Autodesk Fusion 360 part; units mm, degrees
(part 4 of 5)
sketch "Boceto5" plane through (0, 0, 0) normal (0, -1, 0) x (1, 0, 0)
  line L0 (-30, -63.3205) -> (-16, -63.3205)
  line L1 (-16, -63.3205) -> (-16, -68.1205)
  line L2 (-16, -68.1205) -> (-30, -68.1205)
  line L3 (-30, -68.1205) -> (-30, -105)
  line L4 (-30, -105) -> (30, -105)
  line L5 (30, -105) -> (30, -68.1205)
  line L6 (30, -68.1205) -> (16, -68.1205)
  line L7 (16, -68.1205) -> (16, -63.3205)
  line L8 (16, -63.3205) -> (30, -63.3205)
  line L9 (30, -63.3205) -> (30, -62.3205)
  arc A0 (32.0096, -54.8205) -> (30, -62.3205) centre (45, -62.3205) ccw
  line L10 (32.0096, -54.8205) -> (56.4434, -12.5)
  arc A1 (69.4338, -5) -> (56.4434, -12.5) centre (69.4338, -20) ccw
  line L11 (69.4338, -5) -> (101.3943, -5)
  arc A2 (107.5227, -7.8577) -> (101.3943, -5) centre (101.3943, -13) ccw
  line L12 (107.5227, -7.8577) -> (126.7013, -30.7139)
  arc A3 (126.7013, -30.7139) -> (130.5315, -32.5) centre (130.5315, -27.5) ccw
  line L13 (130.5315, -32.5) -> (131.95, -32.5)
  line L14 (131.95, -32.5) -> (133.2, -31.25)
  line L15 (133.2, -31.25) -> (133.2, -5)
  line L16 (133.2, -5) -> (138, -5)
  line L17 (138, -5) -> (138, -31.5)
  line L18 (138, -31.5) -> (139, -32.5)
  line L19 (139, -32.5) -> (141.0289, -32.5)
  arc A4 (141.0289, -32.5) -> (149.6891, -17.5) centre (141.0289, -22.5) ccw
  arc A5 (148.5274, 15.3125) -> (149.6891, -17.5) centre (180, 0) ccw
  arc A6 (148.5274, 15.3125) -> (144.0313, 22.5) centre (144.0313, 17.5) ccw
  line L20 (144.0313, 22.5) -> (131.9209, 22.5)
  arc A7 (131.9209, 22.5) -> (125.7926, 19.6423) centre (131.9209, 14.5) ccw
  line L21 (125.7926, 19.6423) -> (115.9041, 7.8577)
  arc A8 (109.7758, 5) -> (115.9041, 7.8577) centre (109.7758, 13) ccw
  line L22 (109.7758, 5) -> (35, 5)
  arc A9 (30, 10) -> (35, 5) centre (35, 10) ccw
  line L23 (30, 10) -> (30, 12.6048)
  arc A10 (30, 12.6048) -> (26.8657, 15.6018) centre (27, 12.6048) ccw
  arc A11 (22.4813, 15.4213) -> (26.8657, 15.6018) centre (0, 615) ccw
  arc A12 (22.4813, 15.4213) -> (22, 14.9217) centre (22.5, 14.9217) ccw
  line L24 (22, 14.9217) -> (22, 8)
  line L25 (22, 8) -> (17.2, 8)
  line L26 (17.2, 8) -> (17.2, 14.7323)
  arc A13 (17.2, 14.7323) -> (16.6861, 15.2321) centre (16.7, 14.7323) ccw
  arc A14 (10.7514, 15.0963) -> (16.6861, 15.2321) centre (0, 615) ccw
  line L27 (10.7514, 15.0963) -> (6.108, 2.3387)
  arc A15 (0, 11.0618) -> (6.108, 2.3387) centre (0, 4.5618) ccw
  arc A16 (0, 9.0618) -> (0, 11.0618) centre (0, 10.0618) ccw
  arc A17 (0, 9.0618) -> (4.2286, 3.0227) centre (0, 4.5618) ccw
  line L28 (4.2286, 3.0227) -> (8.6105, 15.0618)
  arc A18 (-16.6861, 15.2321) -> (8.6105, 15.0618) centre (0, 615) ccw
  arc A19 (-16.6861, 15.2321) -> (-17.2, 14.7323) centre (-16.7, 14.7323) ccw
  line L29 (-17.2, 14.7323) -> (-17.2, 8)
  line L30 (-17.2, 8) -> (-22, 8)
  line L31 (-22, 8) -> (-22, 14.9217)
  arc A20 (-22, 14.9217) -> (-22.4813, 15.4213) centre (-22.5, 14.9217) ccw
  arc A21 (-26.8657, 15.6018) -> (-22.4813, 15.4213) centre (0, 615) ccw
  arc A22 (-26.8657, 15.6018) -> (-30, 12.6048) centre (-27, 12.6048) ccw
  line L32 (-30, 12.6048) -> (-30, 10)
  arc A23 (-35, 5) -> (-30, 10) centre (-35, 10) ccw
  line L33 (-35, 5) -> (-109.7758, 5)
  arc A24 (-115.9041, 7.8577) -> (-109.7758, 5) centre (-109.7758, 13) ccw
  line L34 (-115.9041, 7.8577) -> (-125.7926, 19.6423)
  arc A25 (-125.7926, 19.6423) -> (-131.9209, 22.5) centre (-131.9209, 14.5) ccw
  line L35 (-131.9209, 22.5) -> (-144.0313, 22.5)
  arc A26 (-144.0313, 22.5) -> (-148.5274, 15.3125) centre (-144.0313, 17.5) ccw
  arc A27 (-149.6891, -17.5) -> (-148.5274, 15.3125) centre (-180, 0) ccw
  arc A28 (-149.6891, -17.5) -> (-141.0289, -32.5) centre (-141.0289, -22.5) ccw
  line L36 (-141.0289, -32.5) -> (-139, -32.5)
  line L37 (-139, -32.5) -> (-138, -31.5)
  line L38 (-138, -31.5) -> (-138, -5)
  line L39 (-138, -5) -> (-133.2, -5)
  line L40 (-133.2, -5) -> (-133.2, -31.25)
  line L41 (-133.2, -31.25) -> (-131.95, -32.5)
  line L42 (-131.95, -32.5) -> (-130.5315, -32.5)
  arc A29 (-130.5315, -32.5) -> (-126.7013, -30.7139) centre (-130.5315, -27.5) ccw
  line L43 (-126.7013, -30.7139) -> (-107.5227, -7.8577)
  arc A30 (-101.3943, -5) -> (-107.5227, -7.8577) centre (-101.3943, -13) ccw
  line L44 (-101.3943, -5) -> (-69.4338, -5)
  arc A31 (-56.4434, -12.5) -> (-69.4338, -5) centre (-69.4338, -20) ccw
  line L45 (-56.4434, -12.5) -> (-32.0096, -54.8205)
  arc A32 (-30, -62.3205) -> (-32.0096, -54.8205) centre (-45, -62.3205) ccw
  line L46 (-30, -62.3205) -> (-30, -63.3205)
  circle A33 centre (-138.0313, 4.5) radius 2.5
  circle A34 centre (140.0313, 14.5) radius 4
  arc A35 (-34.6651, -40.2211) -> (-30, -38.9711) centre (-32.5, -38.9711) ccw
  line L47 (-34.6651, -40.2211) -> (-52.8349, -8.75)
  arc A36 (-50.6699, -5) -> (-52.8349, -8.75) centre (-50.6699, -7.5) ccw
  line L48 (-50.6699, -5) -> (-32.5, -5)
  arc A37 (-30, -7.5) -> (-32.5, -5) centre (-32.5, -7.5) ccw
  line L49 (-30, -7.5) -> (-30, -38.9711)
  arc A38 (-128.2, -19.2264) -> (-124.6679, -20.512) centre (-126.2, -19.2264) ccw
  line L50 (-128.2, -19.2264) -> (-128.2, -7)
  arc A39 (-126.2, -5) -> (-128.2, -7) centre (-126.2, -7) ccw
  line L51 (-126.2, -5) -> (-115.9408, -5)
  arc A40 (-114.4087, -8.2856) -> (-115.9408, -5) centre (-115.9408, -7) ccw
  line L52 (-114.4087, -8.2856) -> (-124.6679, -20.512)
  line L53 (52.8349, -8.75) -> (34.6651, -40.2211)
  arc A41 (30, -38.9711) -> (34.6651, -40.2211) centre (32.5, -38.9711) ccw
  line L54 (30, -38.9711) -> (30, -7.5)
  arc A42 (32.5, -5) -> (30, -7.5) centre (32.5, -7.5) ccw
  line L55 (32.5, -5) -> (50.6699, -5)
  arc A43 (52.8349, -8.75) -> (50.6699, -5) centre (50.6699, -7.5) ccw
  arc A44 (115.9408, -5) -> (114.4087, -8.2856) centre (115.9408, -7) ccw
  line L56 (115.9408, -5) -> (126.2, -5)
  arc A45 (128.2, -7) -> (126.2, -5) centre (126.2, -7) ccw
  line L57 (128.2, -7) -> (128.2, -19.2264)
  arc A46 (124.6679, -20.512) -> (128.2, -19.2264) centre (126.2, -19.2264) ccw
  line L58 (124.6679, -20.512) -> (114.4087, -8.2856)
  circle A47 centre (143.9289, -24) radius 2.5
  arc A48 (-129.934, 16.7992) -> (-131.7, 16.1564) centre (-130.7, 16.1564) ccw
  line L59 (-129.934, 16.7992) -> (-117.2162, 1.6428)
  arc A49 (-117.9823, 0) -> (-117.2162, 1.6428) centre (-117.9823, 1) ccw
  line L60 (-117.9823, 0) -> (-130.7, 0)
  arc A50 (-131.7, 1) -> (-130.7, 0) centre (-130.7, 1) ccw
  line L61 (-131.7, 1) -> (-131.7, 16.1564)
  arc A51 (131.7, 16.1564) -> (129.934, 16.7992) centre (130.7, 16.1564) ccw
  line L62 (131.7, 16.1564) -> (131.7, 1)
  arc A52 (130.7, 0) -> (131.7, 1) centre (130.7, 1) ccw
  line L63 (130.7, 0) -> (117.9823, 0)
  arc A53 (117.2162, 1.6428) -> (117.9823, 0) centre (117.9823, 1) ccw
  line L64 (117.2162, 1.6428) -> (129.934, 16.7992)
  circle A54 centre (-143.9289, -24) radius 2.5
  circle A55 centre (138.0313, 4.5) radius 2.5
  circle A56 centre (-140.0313, 14.5) radius 4
  line L65 (4, -47.2343) -> (4, -38)
  arc A57 (6, -36) -> (4, -38) centre (6, -38) ccw
  line L66 (6, -36) -> (17.005, -36)
  arc A58 (18.2906, -39.5321) -> (17.005, -36) centre (17.005, -38) ccw
  line L67 (18.2906, -39.5321) -> (7.2856, -48.7664)
  arc A59 (4, -47.2343) -> (7.2856, -48.7664) centre (6, -47.2343) ccw
  line L68 (-4, -38) -> (-4, -47.2343)
  arc A60 (-7.2856, -48.7664) -> (-4, -47.2343) centre (-6, -47.2343) ccw
  line L69 (-7.2856, -48.7664) -> (-18.2906, -39.5321)
  arc A61 (-17.005, -36) -> (-18.2906, -39.5321) centre (-17.005, -38) ccw
  line L70 (-17.005, -36) -> (-6, -36)
  arc A62 (-4, -38) -> (-6, -36) centre (-6, -38) ccw
  line L71 (10.6349, -53.7884) -> (19.2144, -46.5894)
  arc A63 (22.5, -48.1215) -> (19.2144, -46.5894) centre (20.5, -48.1215) ccw
  line L72 (22.5, -48.1215) -> (22.5, -55.3205)
  arc A64 (20.5, -57.3205) -> (22.5, -55.3205) centre (20.5, -55.3205) ccw
  line L73 (20.5, -57.3205) -> (11.9205, -57.3205)
  arc A65 (10.6349, -53.7884) -> (11.9205, -57.3205) centre (11.9205, -55.3205) ccw
  line L74 (-16.1716, -5) -> (16.1716, -5)
  arc A66 (17.5858, -5.5858) -> (16.1716, -5) centre (16.1716, -7) ccw
  line L75 (17.5858, -5.5858) -> (20.4142, -8.4142)
  arc A67 (21, -9.8284) -> (20.4142, -8.4142) centre (19, -9.8284) ccw
  line L76 (21, -9.8284) -> (21, -25.1716)
  arc A68 (20.4142, -26.5858) -> (21, -25.1716) centre (19, -25.1716) ccw
  line L77 (20.4142, -26.5858) -> (17.5858, -29.4142)
  arc A69 (16.1716, -30) -> (17.5858, -29.4142) centre (16.1716, -28) ccw
  line L78 (16.1716, -30) -> (-16.1716, -30)
  arc A70 (-17.5858, -29.4142) -> (-16.1716, -30) centre (-16.1716, -28) ccw
  line L79 (-17.5858, -29.4142) -> (-20.4142, -26.5858)
  arc A71 (-21, -25.1716) -> (-20.4142, -26.5858) centre (-19, -25.1716) ccw
  line L80 (-21, -25.1716) -> (-21, -9.8284)
  arc A72 (-20.4142, -8.4142) -> (-21, -9.8284) centre (-19, -9.8284) ccw
  line L81 (-20.4142, -8.4142) -> (-17.5858, -5.5858)
  arc A73 (-16.1716, -5) -> (-17.5858, -5.5858) centre (-16.1716, -7) ccw
  line L82 (-11.9205, -57.3205) -> (-20.5, -57.3205)
  arc A74 (-22.5, -55.3205) -> (-20.5, -57.3205) centre (-20.5, -55.3205) ccw
  line L83 (-22.5, -55.3205) -> (-22.5, -48.1215)
  arc A75 (-19.2144, -46.5894) -> (-22.5, -48.1215) centre (-20.5, -48.1215) ccw
  line L84 (-19.2144, -46.5894) -> (-10.6349, -53.7884)
  arc A76 (-11.9205, -57.3205) -> (-10.6349, -53.7884) centre (-11.9205, -55.3205) ccw
  line L85 (-30, -92.2) -> (-20, -92.2)
  line L86 (-20, -92.2) -> (-20, -97)
  line L87 (-20, -97) -> (-30, -97)
  line L88 (-30, -97) -> (-30, -92.2)
  line L89 (0, -105) -> (0, -63.3205)
  line L90 (-21, -84.2) -> (-21, -78.1205)
  line L91 (-19, -76.1205) -> (-13.0951, -76.1205)
  line L92 (-11.6604, -79.514) -> (-17.5653, -85.5935)
  line L93 (-13.4347, -89.9523) -> (0, -76.1205)
  line L94 (-12, -93.3458) -> (0, -93.3458)
  arc A77 (-21, -84.2) -> (-17.5653, -85.5935) centre (-19, -84.2) ccw
  arc A78 (-11.6604, -79.514) -> (-13.0951, -76.1205) centre (-13.0951, -78.1205) ccw
  arc A79 (-19, -76.1205) -> (-21, -78.1205) centre (-19, -78.1205) ccw
  arc A80 (-13.4347, -89.9523) -> (-12, -93.3458) centre (-12, -91.3458) ccw
  line L95 (0, -63.3205) -> (-5, -63.3205)
  line L96 (-8, -66.3205) -> (-8, -67.1205)
  line L97 (-5, -70.1205) -> (0, -70.1205)
  arc A81 (-5, -63.3205) -> (-8, -66.3205) centre (-5, -66.3205) ccw
  arc A82 (-8, -67.1205) -> (-5, -70.1205) centre (-5, -67.1205) ccw
  line L98 (-30, -97) -> (-30, -101)
  line L99 (-26, -105) -> (-10, -105)
  line L100 (-10, -105) -> (0, -100.3458)
  arc A83 (-30, -101) -> (-26, -105) centre (-26, -101) ccw
  line L101 (10, -105) -> (0, -100.3458)
  line L102 (26, -105) -> (10, -105)
  arc A84 (26, -105) -> (30, -101) centre (26, -101) ccw
  line L103 (12, -93.3458) -> (0, -93.3458)
  arc A85 (12, -93.3458) -> (13.4347, -89.9523) centre (12, -91.3458) ccw
  line L104 (13.4347, -89.9523) -> (0, -76.1205)
  line L105 (30, -92.2) -> (20, -92.2)
  line L106 (20, -92.2) -> (20, -97)
  line L107 (20, -97) -> (30, -97)
  line L108 (30, -97) -> (30, -101)
  line L109 (11.6604, -79.514) -> (17.5653, -85.5935)
  arc A86 (17.5653, -85.5935) -> (21, -84.2) centre (19, -84.2) ccw
  line L110 (21, -84.2) -> (21, -78.1205)
  line L111 (19, -76.1205) -> (13.0951, -76.1205)
  arc A87 (21, -78.1205) -> (19, -76.1205) centre (19, -78.1205) ccw
  arc A88 (13.0951, -76.1205) -> (11.6604, -79.514) centre (13.0951, -78.1205) ccw
  line L112 (5, -70.1205) -> (0, -70.1205)
  arc A89 (5, -70.1205) -> (8, -67.1205) centre (5, -67.1205) ccw
  arc A90 (8, -66.3205) -> (5, -63.3205) centre (5, -66.3205) ccw
  line L113 (8, -66.3205) -> (8, -67.1205)
  line L114 (0, -63.3205) -> (5, -63.3205)
  point P0 (-30, -105)
  dimension "d116" = 10
  dimension "d117" = 4.8
  dimension "d119" = 8
  dimension "d120" = 24.0795
  dimension "d121" = 9
  dimension "d122" = 8
  dimension "d124" = 2
  dimension "d125" = 2
  dimension "d126" = 8
  dimension "d127" = 2
  dimension "d128" = 8
  dimension "d129" = 6
  dimension "d130" = 6
  dimension "d131" = 6
  dimension "d132" = 8
  dimension "d133" = 3
  dimension "d134" = 7
  dimension "d135" = 20
  dimension "d136" = 4
  constraint horizontal L85
  constraint vertical L86
  constraint horizontal L87
  constraint vertical L88
  constraint coincident L3 L85.start
  constraint midpoint L4 L89.start
  constraint perpendicular L4 L89
  constraint parallel L3 L90
  constraint perpendicular L3 L91
  constraint parallel L92 L93
  constraint coincident L89 L93.end
  constraint coincident L89 L94.end
  constraint perpendicular L89 L94
  constraint tangent L90 A77
  constraint tangent L92 A77
  constraint tangent L92 A78
  constraint tangent L91 A78
  constraint equal A77 A78
  constraint tangent L91 A79
  constraint tangent L90 A79
  constraint tangent L93 A80
  constraint tangent L94 A80
  constraint horizontal L95
  constraint perpendicular L95 L96
  constraint coincident L89 L97.end
  constraint perpendicular L89 L97
  constraint tangent L95 A81
  constraint tangent L96 A81
  constraint tangent L97 A82
  constraint tangent L96 A82
  constraint equal A81 A82
  constraint coincident L91 L93.end
  constraint coincident P0 L3.end
  constraint coincident L4 L99.end
  constraint coincident L89 L100.end
  constraint coincident P0 L98
  constraint coincident P0 L99
  constraint tangent L98 A83
  constraint tangent L99 A83
  constraint symmetric L85.start L89 L105.start
  constraint symmetric L85.end L89 L105.end
  constraint symmetric L86.end L89 L106.end
  constraint symmetric L87.end L89 L107.end
  constraint symmetric L89 L93.end L104.end
  constraint symmetric L89 L94.end L103.end
  constraint symmetric L89 L90.start A86.end
  constraint symmetric L89 L92.end L109.end
  constraint symmetric L89 A77 A86
  constraint symmetric L89 L92.start L109.start
  constraint symmetric L89 L91.end L111.end
  constraint symmetric L89 A78 A88
  constraint symmetric L89 L91.start L111.start
  constraint symmetric L89 L90.end L110.end
  constraint symmetric L89 A79 A87
  constraint symmetric L89 L93.start A85.end
  constraint symmetric L89 L94.start L103.start
  constraint symmetric L89 A80 A85
  constraint symmetric L89 L95.start L114.start
  constraint symmetric L89 L97.end L112.end
  constraint symmetric L89 L95.end A90.end
  constraint symmetric L89 L96.start A90.start
  constraint symmetric L89 A81 A90
  constraint symmetric L89 L97.start L112.start
  constraint symmetric L89 L96.end A89.end
  constraint symmetric L89 A82 A89
  constraint symmetric L89 L99.end L101.start
  constraint symmetric L89 L100.end L101.end
  constraint symmetric L89 L98.end A84.end
  constraint symmetric L89 L99.start L102.start
  constraint symmetric L89 A83 A84
  measures "d116" distance of L85.start L85.end
  measures "d117" distance of L85.start L87.end
  measures "d119" distance of L4 L87
  measures "d120" distance of L2 L85
  measures "d121" distance of L3 L90
  measures "d122" distance of L2 L91
  measures "d124" radius of A77
  measures "d125" radius of A79
  measures "d126" vertical distance of L85.end A77.centre
  measures "d127" radius of A80
  measures "d128" distance of L86 A80.centre
  measures "d129" distance of L92 L93
  measures "d130" distance of L82 L95
  measures "d131" distance of L91 L97
  measures "d132" distance of L1 L96
  measures "d133" radius of A81
  measures "d134" distance of L94 L100.end
  measures "d135" distance of P0 L99.end
  measures "d136" radius of A83
extrude "Extruir4" cut sketch "Boceto5" against normal blind 4.8 contours L3 L85 L86 L87 L88 | L3 L4 A83 | L4 L89 L100 | L4 L89 L101 | L4 L5 A84 | L5 L105 L106 L107 | L89 L93 L94 A80 | L89 L103 A85 L104 | L89 L95 L96 L97 A81 A82 | L89 L112 A89 A90 L113 L114 | L90 L91 L92 A77 A78 A79 | L109 A86 L110 L111 A87 A88
fillet "Empalme4" radius 2 2 edges at (0, 2.4, -76.1205) (0, 2.4, -100.3458)
sketch "Boceto7" plane through (0, 0, 0) normal (0, -1, 0) x (1, 0, 0)
  arc A0 (-30, -101) -> (-26, -105) centre (-26, -101) ccw
  line L0 (-26, -105) -> (-10, -105)
  line L1 (-10, -105) -> (-0.8439, -100.7385)
  arc A1 (0.8439, -100.7385) -> (-0.8439, -100.7385) centre (0, -102.5518) ccw
  line L2 (0.8439, -100.7385) -> (10, -105)
  line L3 (10, -105) -> (26, -105)
  arc A2 (26, -105) -> (30, -101) centre (26, -101) ccw
  line L4 (30, -101) -> (30, -97)
  line L5 (30, -97) -> (20, -97)
  line L6 (20, -97) -> (20, -92.2)
  line L7 (20, -92.2) -> (30, -92.2)
  line L8 (30, -92.2) -> (30, -68.1205)
  line L9 (30, -68.1205) -> (16, -68.1205)
  line L10 (16, -68.1205) -> (16, -63.3205)
  line L11 (16, -63.3205) -> (30, -63.3205)
  line L12 (30, -63.3205) -> (30, -62.3205)
  arc A3 (32.0096, -54.8205) -> (30, -62.3205) centre (45, -62.3205) ccw
  line L13 (32.0096, -54.8205) -> (56.4434, -12.5)
  arc A4 (69.4338, -5) -> (56.4434, -12.5) centre (69.4338, -20) ccw
  line L14 (69.4338, -5) -> (101.3943, -5)
  arc A5 (107.5227, -7.8577) -> (101.3943, -5) centre (101.3943, -13) ccw
  line L15 (107.5227, -7.8577) -> (126.7013, -30.7139)
  arc A6 (126.7013, -30.7139) -> (130.5315, -32.5) centre (130.5315, -27.5) ccw
  line L16 (130.5315, -32.5) -> (131.95, -32.5)
  line L17 (131.95, -32.5) -> (133.2, -31.25)
  line L18 (133.2, -31.25) -> (133.2, -5)
  line L19 (133.2, -5) -> (138, -5)
  line L20 (138, -5) -> (138, -31.5)
  line L21 (138, -31.5) -> (139, -32.5)
  line L22 (139, -32.5) -> (141.0289, -32.5)
  arc A7 (141.0289, -32.5) -> (149.6891, -17.5) centre (141.0289, -22.5) ccw
  arc A8 (148.5274, 15.3125) -> (149.6891, -17.5) centre (180, 0) ccw
  arc A9 (148.5274, 15.3125) -> (144.0313, 22.5) centre (144.0313, 17.5) ccw
  line L23 (144.0313, 22.5) -> (131.9209, 22.5)
  arc A10 (131.9209, 22.5) -> (125.7926, 19.6423) centre (131.9209, 14.5) ccw
  line L24 (125.7926, 19.6423) -> (115.9041, 7.8577)
  arc A11 (109.7758, 5) -> (115.9041, 7.8577) centre (109.7758, 13) ccw
  line L25 (109.7758, 5) -> (35, 5)
  arc A12 (30, 10) -> (35, 5) centre (35, 10) ccw
  line L26 (30, 10) -> (30, 12.6048)
  arc A13 (30, 12.6048) -> (26.8657, 15.6018) centre (27, 12.6048) ccw
  arc A14 (22.4813, 15.4213) -> (26.8657, 15.6018) centre (0, 615) ccw
  arc A15 (22.4813, 15.4213) -> (22, 14.9217) centre (22.5, 14.9217) ccw
  line L27 (22, 14.9217) -> (22, 8)
  line L28 (22, 8) -> (17.2, 8)
  line L29 (17.2, 8) -> (17.2, 14.7323)
  arc A16 (17.2, 14.7323) -> (16.6861, 15.2321) centre (16.7, 14.7323) ccw
  arc A17 (10.7514, 15.0963) -> (16.6861, 15.2321) centre (0, 615) ccw
  line L30 (10.7514, 15.0963) -> (6.108, 2.3387)
  arc A18 (0, 11.0618) -> (6.108, 2.3387) centre (0, 4.5618) ccw
  arc A19 (0, 9.0618) -> (0, 11.0618) centre (0, 10.0618) ccw
  arc A20 (0, 9.0618) -> (4.2286, 3.0227) centre (0, 4.5618) ccw
  line L31 (4.2286, 3.0227) -> (8.6105, 15.0618)
  arc A21 (-16.6861, 15.2321) -> (8.6105, 15.0618) centre (0, 615) ccw
  arc A22 (-16.6861, 15.2321) -> (-17.2, 14.7323) centre (-16.7, 14.7323) ccw
  line L32 (-17.2, 14.7323) -> (-17.2, 8)
  line L33 (-17.2, 8) -> (-22, 8)
  line L34 (-22, 8) -> (-22, 14.9217)
  arc A23 (-22, 14.9217) -> (-22.4813, 15.4213) centre (-22.5, 14.9217) ccw
  arc A24 (-26.8657, 15.6018) -> (-22.4813, 15.4213) centre (0, 615) ccw
  arc A25 (-26.8657, 15.6018) -> (-30, 12.6048) centre (-27, 12.6048) ccw
  line L35 (-30, 12.6048) -> (-30, 10)
  arc A26 (-35, 5) -> (-30, 10) centre (-35, 10) ccw
  line L36 (-35, 5) -> (-109.7758, 5)
  arc A27 (-115.9041, 7.8577) -> (-109.7758, 5) centre (-109.7758, 13) ccw
  line L37 (-115.9041, 7.8577) -> (-125.7926, 19.6423)
  arc A28 (-125.7926, 19.6423) -> (-131.9209, 22.5) centre (-131.9209, 14.5) ccw
  line L38 (-131.9209, 22.5) -> (-144.0313, 22.5)
  arc A29 (-144.0313, 22.5) -> (-148.5274, 15.3125) centre (-144.0313, 17.5) ccw
  arc A30 (-149.6891, -17.5) -> (-148.5274, 15.3125) centre (-180, 0) ccw
  arc A31 (-149.6891, -17.5) -> (-141.0289, -32.5) centre (-141.0289, -22.5) ccw
  line L39 (-141.0289, -32.5) -> (-139, -32.5)
  line L40 (-139, -32.5) -> (-138, -31.5)
  line L41 (-138, -31.5) -> (-138, -5)
  line L42 (-138, -5) -> (-133.2, -5)
  line L43 (-133.2, -5) -> (-133.2, -31.25)
  line L44 (-133.2, -31.25) -> (-131.95, -32.5)
  line L45 (-131.95, -32.5) -> (-130.5315, -32.5)
  arc A32 (-130.5315, -32.5) -> (-126.7013, -30.7139) centre (-130.5315, -27.5) ccw
  line L46 (-126.7013, -30.7139) -> (-107.5227, -7.8577)
  arc A33 (-101.3943, -5) -> (-107.5227, -7.8577) centre (-101.3943, -13) ccw
  line L47 (-101.3943, -5) -> (-69.4338, -5)
  arc A34 (-56.4434, -12.5) -> (-69.4338, -5) centre (-69.4338, -20) ccw
  line L48 (-56.4434, -12.5) -> (-32.0096, -54.8205)
  arc A35 (-30, -62.3205) -> (-32.0096, -54.8205) centre (-45, -62.3205) ccw
  line L49 (-30, -62.3205) -> (-30, -63.3205)
  line L50 (-30, -63.3205) -> (-16, -63.3205)
  line L51 (-16, -63.3205) -> (-16, -68.1205)
  line L52 (-16, -68.1205) -> (-30, -68.1205)
  line L53 (-30, -68.1205) -> (-30, -92.2)
  line L54 (-30, -92.2) -> (-20, -92.2)
  line L55 (-20, -92.2) -> (-20, -97)
  line L56 (-20, -97) -> (-30, -97)
  line L57 (-30, -97) -> (-30, -101)
  line L58 (-11.9205, -57.3205) -> (-20.5, -57.3205)
  arc A36 (-22.5, -55.3205) -> (-20.5, -57.3205) centre (-20.5, -55.3205) ccw
  line L59 (-22.5, -55.3205) -> (-22.5, -48.1215)
  arc A37 (-19.2144, -46.5894) -> (-22.5, -48.1215) centre (-20.5, -48.1215) ccw
  line L60 (-19.2144, -46.5894) -> (-10.6349, -53.7884)
  arc A38 (-11.9205, -57.3205) -> (-10.6349, -53.7884) centre (-11.9205, -55.3205) ccw
  line L61 (-16.1716, -5) -> (16.1716, -5)
  arc A39 (17.5858, -5.5858) -> (16.1716, -5) centre (16.1716, -7) ccw
  line L62 (17.5858, -5.5858) -> (20.4142, -8.4142)
  arc A40 (21, -9.8284) -> (20.4142, -8.4142) centre (19, -9.8284) ccw
  line L63 (21, -9.8284) -> (21, -25.1716)
  arc A41 (20.4142, -26.5858) -> (21, -25.1716) centre (19, -25.1716) ccw
  line L64 (20.4142, -26.5858) -> (17.5858, -29.4142)
  arc A42 (16.1716, -30) -> (17.5858, -29.4142) centre (16.1716, -28) ccw
  line L65 (16.1716, -30) -> (-16.1716, -30)
  arc A43 (-17.5858, -29.4142) -> (-16.1716, -30) centre (-16.1716, -28) ccw
  line L66 (-17.5858, -29.4142) -> (-20.4142, -26.5858)
  arc A44 (-21, -25.1716) -> (-20.4142, -26.5858) centre (-19, -25.1716) ccw
  line L67 (-21, -25.1716) -> (-21, -9.8284)
  arc A45 (-20.4142, -8.4142) -> (-21, -9.8284) centre (-19, -9.8284) ccw
  line L68 (-20.4142, -8.4142) -> (-17.5858, -5.5858)
  arc A46 (-16.1716, -5) -> (-17.5858, -5.5858) centre (-16.1716, -7) ccw
  line L69 (10.6349, -53.7884) -> (19.2144, -46.5894)
  arc A47 (22.5, -48.1215) -> (19.2144, -46.5894) centre (20.5, -48.1215) ccw
  line L70 (22.5, -48.1215) -> (22.5, -55.3205)
  arc A48 (20.5, -57.3205) -> (22.5, -55.3205) centre (20.5, -55.3205) ccw
  line L71 (20.5, -57.3205) -> (11.9205, -57.3205)
  arc A49 (10.6349, -53.7884) -> (11.9205, -57.3205) centre (11.9205, -55.3205) ccw
  line L72 (-4, -38) -> (-4, -47.2343)
  arc A50 (-7.2856, -48.7664) -> (-4, -47.2343) centre (-6, -47.2343) ccw
  line L73 (-7.2856, -48.7664) -> (-18.2906, -39.5321)
  arc A51 (-17.005, -36) -> (-18.2906, -39.5321) centre (-17.005, -38) ccw
  line L74 (-17.005, -36) -> (-6, -36)
  arc A52 (-4, -38) -> (-6, -36) centre (-6, -38) ccw
  line L75 (4, -47.2343) -> (4, -38)
  arc A53 (6, -36) -> (4, -38) centre (6, -38) ccw
  line L76 (6, -36) -> (17.005, -36)
  arc A54 (18.2906, -39.5321) -> (17.005, -36) centre (17.005, -38) ccw
  line L77 (18.2906, -39.5321) -> (7.2856, -48.7664)
  arc A55 (4, -47.2343) -> (7.2856, -48.7664) centre (6, -47.2343) ccw
  circle A56 centre (-140.0313, 14.5) radius 4
  circle A57 centre (138.0313, 4.5) radius 2.5
  circle A58 centre (-143.9289, -24) radius 2.5
  arc A59 (131.7, 16.1564) -> (129.934, 16.7992) centre (130.7, 16.1564) ccw
  line L78 (131.7, 16.1564) -> (131.7, 1)
  arc A60 (130.7, 0) -> (131.7, 1) centre (130.7, 1) ccw
  line L79 (130.7, 0) -> (117.9823, 0)
  arc A61 (117.2162, 1.6428) -> (117.9823, 0) centre (117.9823, 1) ccw
  line L80 (117.2162, 1.6428) -> (129.934, 16.7992)
  arc A62 (-129.934, 16.7992) -> (-131.7, 16.1564) centre (-130.7, 16.1564) ccw
  line L81 (-129.934, 16.7992) -> (-117.2162, 1.6428)
  arc A63 (-117.9823, 0) -> (-117.2162, 1.6428) centre (-117.9823, 1) ccw
  line L82 (-117.9823, 0) -> (-130.7, 0)
  arc A64 (-131.7, 1) -> (-130.7, 0) centre (-130.7, 1) ccw
  line L83 (-131.7, 1) -> (-131.7, 16.1564)
  circle A65 centre (143.9289, -24) radius 2.5
  arc A66 (115.9408, -5) -> (114.4087, -8.2856) centre (115.9408, -7) ccw
  line L84 (115.9408, -5) -> (126.2, -5)
  arc A67 (128.2, -7) -> (126.2, -5) centre (126.2, -7) ccw
  line L85 (128.2, -7) -> (128.2, -19.2264)
  arc A68 (124.6679, -20.512) -> (128.2, -19.2264) centre (126.2, -19.2264) ccw
  line L86 (124.6679, -20.512) -> (114.4087, -8.2856)
  line L87 (52.8349, -8.75) -> (34.6651, -40.2211)
  arc A69 (30, -38.9711) -> (34.6651, -40.2211) centre (32.5, -38.9711) ccw
  line L88 (30, -38.9711) -> (30, -7.5)
  arc A70 (32.5, -5) -> (30, -7.5) centre (32.5, -7.5) ccw
  line L89 (32.5, -5) -> (50.6699, -5)
  arc A71 (52.8349, -8.75) -> (50.6699, -5) centre (50.6699, -7.5) ccw
  arc A72 (-128.2, -19.2264) -> (-124.6679, -20.512) centre (-126.2, -19.2264) ccw
  line L90 (-128.2, -19.2264) -> (-128.2, -7)
  arc A73 (-126.2, -5) -> (-128.2, -7) centre (-126.2, -7) ccw
  line L91 (-126.2, -5) -> (-115.9408, -5)
  arc A74 (-114.4087, -8.2856) -> (-115.9408, -5) centre (-115.9408, -7) ccw
  line L92 (-114.4087, -8.2856) -> (-124.6679, -20.512)
  arc A75 (-34.6651, -40.2211) -> (-30, -38.9711) centre (-32.5, -38.9711) ccw
  line L93 (-34.6651, -40.2211) -> (-52.8349, -8.75)
  arc A76 (-50.6699, -5) -> (-52.8349, -8.75) centre (-50.6699, -7.5) ccw
  line L94 (-50.6699, -5) -> (-32.5, -5)
  arc A77 (-30, -7.5) -> (-32.5, -5) centre (-32.5, -7.5) ccw
  line L95 (-30, -7.5) -> (-30, -38.9711)
  circle A78 centre (140.0313, 14.5) radius 4
  circle A79 centre (-138.0313, 4.5) radius 2.5
  line L96 (-8, -67.1205) -> (-8, -66.3205)
  arc A80 (-5, -63.3205) -> (-8, -66.3205) centre (-5, -66.3205) ccw
  line L97 (-5, -63.3205) -> (5, -63.3205)
  arc A81 (8, -66.3205) -> (5, -63.3205) centre (5, -66.3205) ccw
  line L98 (8, -66.3205) -> (8, -67.1205)
  arc A82 (5, -70.1205) -> (8, -67.1205) centre (5, -67.1205) ccw
  line L99 (5, -70.1205) -> (-5, -70.1205)
  arc A83 (-8, -67.1205) -> (-5, -70.1205) centre (-5, -67.1205) ccw
  line L100 (17.5653, -85.5935) -> (11.6604, -79.514)
  arc A84 (13.0951, -76.1205) -> (11.6604, -79.514) centre (13.0951, -78.1205) ccw
  line L101 (13.0951, -76.1205) -> (19, -76.1205)
  arc A85 (21, -78.1205) -> (19, -76.1205) centre (19, -78.1205) ccw
  line L102 (21, -78.1205) -> (21, -84.2)
  arc A86 (17.5653, -85.5935) -> (21, -84.2) centre (19, -84.2) ccw
  line L103 (-19, -76.1205) -> (-13.0951, -76.1205)
  arc A87 (-11.6604, -79.514) -> (-13.0951, -76.1205) centre (-13.0951, -78.1205) ccw
  line L104 (-11.6604, -79.514) -> (-17.5653, -85.5935)
  arc A88 (-21, -84.2) -> (-17.5653, -85.5935) centre (-19, -84.2) ccw
  line L105 (-21, -84.2) -> (-21, -78.1205)
  arc A89 (-19, -76.1205) -> (-21, -78.1205) centre (-19, -78.1205) ccw
  line L106 (1.4347, -77.5976) -> (13.4347, -89.9523)
  arc A90 (12, -93.3458) -> (13.4347, -89.9523) centre (12, -91.3458) ccw
  line L107 (12, -93.3458) -> (-12, -93.3458)
  arc A91 (-13.4347, -89.9523) -> (-12, -93.3458) centre (-12, -91.3458) ccw
  line L108 (-13.4347, -89.9523) -> (-1.4347, -77.5976)
  arc A92 (1.4347, -77.5976) -> (-1.4347, -77.5976) centre (0, -78.991) ccw
  line L109 (117.7113, -20) -> (30, -83.5555)
  line L110 (122.2222, -25.3759) -> (30, -92.2)
  line L111 (0, 1.75) -> (0, 22.5)
  line L112 (-122.2222, -25.3759) -> (-30, -92.2)
  line L113 (-117.7113, -20) -> (-30, -83.5555)
  dimension "d141" = 7
  dimension "d142" = 15
  constraint coincident L15 L109.start
  constraint coincident L15 L110.start
  constraint parallel L109 L110
  constraint symmetric L109.start L111 L113.start
  constraint symmetric L109.end L111 L113.end
  constraint symmetric L110.start L111 L112.start
  constraint symmetric L7.end L111 L53.end
  constraint coincident L8 L7.end
  constraint coincident L8 L109.end
  constraint coincident L7.end L8.start
  constraint coincident L11.end L12.start
  measures "d141" distance of L109 L110
  measures "d142" distance of L84 L109.start
extrude "Extruir6" add sketch "Boceto7" against normal blind 4.8 contours L46 L53 L112 L113 | L8 L15 L109 L110
sketch "Boceto8" plane through (0, 4.8, 0) normal (0, 1, 0) x (-1, 0, 0)
  line L0 (30, -83.5555) -> (30, -68.1205)
  line L1 (30, -68.1205) -> (16, -68.1205)
  line L2 (16, -68.1205) -> (16, -63.3205)
  line L3 (16, -63.3205) -> (30, -63.3205)
  line L4 (30, -63.3205) -> (30, -62.3205)
  arc A0 (32.0096, -54.8205) -> (30, -62.3205) centre (45, -62.3205) ccw
  line L5 (32.0096, -54.8205) -> (56.4434, -12.5)
  arc A1 (69.4338, -5) -> (56.4434, -12.5) centre (69.4338, -20) ccw
  line L6 (69.4338, -5) -> (101.3943, -5)
  arc A2 (107.5227, -7.8577) -> (101.3943, -5) centre (101.3943, -13) ccw
  line L7 (107.5227, -7.8577) -> (117.7113, -20)
  line L8 (117.7113, -20) -> (30, -83.5555)
  line L9 (30, -92.2) -> (122.2222, -25.3759)
  line L10 (122.2222, -25.3759) -> (126.7013, -30.7139)
  arc A3 (126.7013, -30.7139) -> (130.5315, -32.5) centre (130.5315, -27.5) ccw
  line L11 (130.5315, -32.5) -> (131.95, -32.5)
  line L12 (131.95, -32.5) -> (133.2, -31.25)
  line L13 (133.2, -31.25) -> (133.2, -5)
  line L14 (133.2, -5) -> (138, -5)
  line L15 (138, -5) -> (138, -31.5)
  line L16 (138, -31.5) -> (139, -32.5)
  line L17 (139, -32.5) -> (141.0289, -32.5)
  arc A4 (141.0289, -32.5) -> (149.6891, -17.5) centre (141.0289, -22.5) ccw
  arc A5 (148.5274, 15.3125) -> (149.6891, -17.5) centre (180, 0) ccw
  arc A6 (148.5274, 15.3125) -> (144.0313, 22.5) centre (144.0313, 17.5) ccw
  line L18 (144.0313, 22.5) -> (131.9209, 22.5)
  arc A7 (131.9209, 22.5) -> (125.7926, 19.6423) centre (131.9209, 14.5) ccw
  line L19 (125.7926, 19.6423) -> (115.9041, 7.8577)
  arc A8 (109.7758, 5) -> (115.9041, 7.8577) centre (109.7758, 13) ccw
  line L20 (109.7758, 5) -> (35, 5)
  arc A9 (30, 10) -> (35, 5) centre (35, 10) ccw
  line L21 (30, 10) -> (30, 12.6048)
  arc A10 (30, 12.6048) -> (26.8657, 15.6018) centre (27, 12.6048) ccw
  arc A11 (22.4813, 15.4213) -> (26.8657, 15.6018) centre (0, 615) ccw
  arc A12 (22.4813, 15.4213) -> (22, 14.9217) centre (22.5, 14.9217) ccw
  line L22 (22, 14.9217) -> (22, 8)
  line L23 (22, 8) -> (17.2, 8)
  line L24 (17.2, 8) -> (17.2, 14.7323)
  arc A13 (17.2, 14.7323) -> (16.6861, 15.2321) centre (16.7, 14.7323) ccw
  arc A14 (-8.6105, 15.0618) -> (16.6861, 15.2321) centre (0, 615) ccw
  line L25 (-8.6105, 15.0618) -> (-4.2286, 3.0227)
  arc A15 (-4.2286, 3.0227) -> (0, 9.0618) centre (0, 4.5618) ccw
  arc A16 (0, 11.0618) -> (0, 9.0618) centre (0, 10.0618) ccw
  arc A17 (-6.108, 2.3387) -> (0, 11.0618) centre (0, 4.5618) ccw
  line L26 (-6.108, 2.3387) -> (-10.7514, 15.0963)
  arc A18 (-16.6861, 15.2321) -> (-10.7514, 15.0963) centre (0, 615) ccw
  arc A19 (-16.6861, 15.2321) -> (-17.2, 14.7323) centre (-16.7, 14.7323) ccw
  line L27 (-17.2, 14.7323) -> (-17.2, 8)
  line L28 (-17.2, 8) -> (-22, 8)
  line L29 (-22, 8) -> (-22, 14.9217)
  arc A20 (-22, 14.9217) -> (-22.4813, 15.4213) centre (-22.5, 14.9217) ccw
  arc A21 (-26.8657, 15.6018) -> (-22.4813, 15.4213) centre (0, 615) ccw
  arc A22 (-26.8657, 15.6018) -> (-30, 12.6048) centre (-27, 12.6048) ccw
  line L30 (-30, 12.6048) -> (-30, 10)
  arc A23 (-35, 5) -> (-30, 10) centre (-35, 10) ccw
  line L31 (-35, 5) -> (-109.7758, 5)
  arc A24 (-115.9041, 7.8577) -> (-109.7758, 5) centre (-109.7758, 13) ccw
  line L32 (-115.9041, 7.8577) -> (-125.7926, 19.6423)
  arc A25 (-125.7926, 19.6423) -> (-131.9209, 22.5) centre (-131.9209, 14.5) ccw
  line L33 (-131.9209, 22.5) -> (-144.0313, 22.5)
  arc A26 (-144.0313, 22.5) -> (-148.5274, 15.3125) centre (-144.0313, 17.5) ccw
  arc A27 (-149.6891, -17.5) -> (-148.5274, 15.3125) centre (-180, 0) ccw
  arc A28 (-149.6891, -17.5) -> (-141.0289, -32.5) centre (-141.0289, -22.5) ccw
  line L34 (-141.0289, -32.5) -> (-139, -32.5)
  line L35 (-139, -32.5) -> (-138, -31.5)
  line L36 (-138, -31.5) -> (-138, -5)
  line L37 (-138, -5) -> (-133.2, -5)
  line L38 (-133.2, -5) -> (-133.2, -31.25)
  line L39 (-133.2, -31.25) -> (-131.95, -32.5)
  line L40 (-131.95, -32.5) -> (-130.5315, -32.5)
  arc A29 (-130.5315, -32.5) -> (-126.7013, -30.7139) centre (-130.5315, -27.5) ccw
  line L41 (-126.7013, -30.7139) -> (-122.2222, -25.3759)
  line L42 (-122.2222, -25.3759) -> (-30, -92.2)
  line L43 (-30, -92.2) -> (-20, -92.2)
  line L44 (-20, -92.2) -> (-20, -97)
  line L45 (-20, -97) -> (-30, -97)
  line L46 (-30, -97) -> (-30, -101)
  arc A30 (-30, -101) -> (-26, -105) centre (-26, -101) ccw
  line L47 (-26, -105) -> (-10, -105)
  line L48 (-10, -105) -> (-0.8439, -100.7385)
  arc A31 (0.8439, -100.7385) -> (-0.8439, -100.7385) centre (0, -102.5518) ccw
  line L49 (0.8439, -100.7385) -> (10, -105)
  line L50 (10, -105) -> (26, -105)
  arc A32 (26, -105) -> (30, -101) centre (26, -101) ccw
  line L51 (30, -101) -> (30, -97)
  line L52 (30, -97) -> (20, -97)
  line L53 (20, -97) -> (20, -92.2)
  line L54 (20, -92.2) -> (30, -92.2)
  line L55 (-30, -83.5555) -> (-117.7113, -20)
  line L56 (-117.7113, -20) -> (-107.5227, -7.8577)
  arc A33 (-101.3943, -5) -> (-107.5227, -7.8577) centre (-101.3943, -13) ccw
  line L57 (-101.3943, -5) -> (-69.4338, -5)
  arc A34 (-56.4434, -12.5) -> (-69.4338, -5) centre (-69.4338, -20) ccw
  line L58 (-56.4434, -12.5) -> (-32.0096, -54.8205)
  arc A35 (-30, -62.3205) -> (-32.0096, -54.8205) centre (-45, -62.3205) ccw
  line L59 (-30, -62.3205) -> (-30, -63.3205)
  line L60 (-30, -63.3205) -> (-16, -63.3205)
  line L61 (-16, -63.3205) -> (-16, -68.1205)
  line L62 (-16, -68.1205) -> (-30, -68.1205)
  line L63 (-30, -68.1205) -> (-30, -83.5555)
  line L64 (20.5, -57.3205) -> (11.9205, -57.3205)
  arc A36 (10.6349, -53.7884) -> (11.9205, -57.3205) centre (11.9205, -55.3205) ccw
  line L65 (10.6349, -53.7884) -> (19.2144, -46.5894)
  arc A37 (22.5, -48.1215) -> (19.2144, -46.5894) centre (20.5, -48.1215) ccw
  line L66 (22.5, -48.1215) -> (22.5, -55.3205)
  arc A38 (20.5, -57.3205) -> (22.5, -55.3205) centre (20.5, -55.3205) ccw
  line L67 (-16.1716, -5) -> (16.1716, -5)
  arc A39 (17.5858, -5.5858) -> (16.1716, -5) centre (16.1716, -7) ccw
  line L68 (17.5858, -5.5858) -> (20.4142, -8.4142)
  arc A40 (21, -9.8284) -> (20.4142, -8.4142) centre (19, -9.8284) ccw
  line L69 (21, -9.8284) -> (21, -25.1716)
  arc A41 (20.4142, -26.5858) -> (21, -25.1716) centre (19, -25.1716) ccw
  line L70 (20.4142, -26.5858) -> (17.5858, -29.4142)
  arc A42 (16.1716, -30) -> (17.5858, -29.4142) centre (16.1716, -28) ccw
  line L71 (16.1716, -30) -> (-16.1716, -30)
  arc A43 (-17.5858, -29.4142) -> (-16.1716, -30) centre (-16.1716, -28) ccw
  line L72 (-17.5858, -29.4142) -> (-20.4142, -26.5858)
  arc A44 (-21, -25.1716) -> (-20.4142, -26.5858) centre (-19, -25.1716) ccw
  line L73 (-21, -25.1716) -> (-21, -9.8284)
  arc A45 (-20.4142, -8.4142) -> (-21, -9.8284) centre (-19, -9.8284) ccw
  line L74 (-20.4142, -8.4142) -> (-17.5858, -5.5858)
  arc A46 (-16.1716, -5) -> (-17.5858, -5.5858) centre (-16.1716, -7) ccw
  line L75 (-19.2144, -46.5894) -> (-10.6349, -53.7884)
  arc A47 (-11.9205, -57.3205) -> (-10.6349, -53.7884) centre (-11.9205, -55.3205) ccw
  line L76 (-11.9205, -57.3205) -> (-20.5, -57.3205)
  arc A48 (-22.5, -55.3205) -> (-20.5, -57.3205) centre (-20.5, -55.3205) ccw
  line L77 (-22.5, -55.3205) -> (-22.5, -48.1215)
  arc A49 (-19.2144, -46.5894) -> (-22.5, -48.1215) centre (-20.5, -48.1215) ccw
  line L78 (4, -47.2343) -> (4, -38)
  arc A50 (6, -36) -> (4, -38) centre (6, -38) ccw
  line L79 (6, -36) -> (17.005, -36)
  arc A51 (18.2906, -39.5321) -> (17.005, -36) centre (17.005, -38) ccw
  line L80 (18.2906, -39.5321) -> (7.2856, -48.7664)
  arc A52 (4, -47.2343) -> (7.2856, -48.7664) centre (6, -47.2343) ccw
  line L81 (-4, -38) -> (-4, -47.2343)
  arc A53 (-7.2856, -48.7664) -> (-4, -47.2343) centre (-6, -47.2343) ccw
  line L82 (-7.2856, -48.7664) -> (-18.2906, -39.5321)
  arc A54 (-17.005, -36) -> (-18.2906, -39.5321) centre (-17.005, -38) ccw
  line L83 (-17.005, -36) -> (-6, -36)
  arc A55 (-4, -38) -> (-6, -36) centre (-6, -38) ccw
  circle A56 centre (140.0313, 14.5) radius 4
  circle A57 centre (-138.0313, 4.5) radius 2.5
  circle A58 centre (143.9289, -24) radius 2.5
  arc A59 (-129.934, 16.7992) -> (-131.7, 16.1564) centre (-130.7, 16.1564) ccw
  line L84 (-129.934, 16.7992) -> (-117.2162, 1.6428)
  arc A60 (-117.9823, 0) -> (-117.2162, 1.6428) centre (-117.9823, 1) ccw
  line L85 (-117.9823, 0) -> (-130.7, 0)
  arc A61 (-131.7, 1) -> (-130.7, 0) centre (-130.7, 1) ccw
  line L86 (-131.7, 1) -> (-131.7, 16.1564)
  arc A62 (131.7, 16.1564) -> (129.934, 16.7992) centre (130.7, 16.1564) ccw
  line L87 (131.7, 16.1564) -> (131.7, 1)
  arc A63 (130.7, 0) -> (131.7, 1) centre (130.7, 1) ccw
  line L88 (130.7, 0) -> (117.9823, 0)
  arc A64 (117.2162, 1.6428) -> (117.9823, 0) centre (117.9823, 1) ccw
  line L89 (117.2162, 1.6428) -> (129.934, 16.7992)
  circle A65 centre (-143.9289, -24) radius 2.5
  arc A66 (-114.4087, -8.2856) -> (-115.9408, -5) centre (-115.9408, -7) ccw
  line L90 (-114.4087, -8.2856) -> (-124.6679, -20.512)
  arc A67 (-128.2, -19.2264) -> (-124.6679, -20.512) centre (-126.2, -19.2264) ccw
  line L91 (-128.2, -19.2264) -> (-128.2, -7)
  arc A68 (-126.2, -5) -> (-128.2, -7) centre (-126.2, -7) ccw
  line L92 (-126.2, -5) -> (-115.9408, -5)
  line L93 (-34.6651, -40.2211) -> (-52.8349, -8.75)
  arc A69 (-50.6699, -5) -> (-52.8349, -8.75) centre (-50.6699, -7.5) ccw
  line L94 (-50.6699, -5) -> (-32.5, -5)
  arc A70 (-30, -7.5) -> (-32.5, -5) centre (-32.5, -7.5) ccw
  line L95 (-30, -7.5) -> (-30, -38.9711)
  arc A71 (-34.6651, -40.2211) -> (-30, -38.9711) centre (-32.5, -38.9711) ccw
  arc A72 (124.6679, -20.512) -> (128.2, -19.2264) centre (126.2, -19.2264) ccw
  line L96 (124.6679, -20.512) -> (114.4087, -8.2856)
  arc A73 (115.9408, -5) -> (114.4087, -8.2856) centre (115.9408, -7) ccw
  line L97 (115.9408, -5) -> (126.2, -5)
  arc A74 (128.2, -7) -> (126.2, -5) centre (126.2, -7) ccw
  line L98 (128.2, -7) -> (128.2, -19.2264)
  arc A75 (30, -38.9711) -> (34.6651, -40.2211) centre (32.5, -38.9711) ccw
  line L99 (30, -38.9711) -> (30, -7.5)
  arc A76 (32.5, -5) -> (30, -7.5) centre (32.5, -7.5) ccw
  line L100 (32.5, -5) -> (50.6699, -5)
  arc A77 (52.8349, -8.75) -> (50.6699, -5) centre (50.6699, -7.5) ccw
  line L101 (52.8349, -8.75) -> (34.6651, -40.2211)
  circle A78 centre (-140.0313, 14.5) radius 4
  circle A79 centre (138.0313, 4.5) radius 2.5
  line L102 (8, -66.3205) -> (8, -67.1205)
  arc A80 (5, -70.1205) -> (8, -67.1205) centre (5, -67.1205) ccw
  line L103 (5, -70.1205) -> (-5, -70.1205)
  arc A81 (-8, -67.1205) -> (-5, -70.1205) centre (-5, -67.1205) ccw
  line L104 (-8, -67.1205) -> (-8, -66.3205)
  arc A82 (-5, -63.3205) -> (-8, -66.3205) centre (-5, -66.3205) ccw
  line L105 (-5, -63.3205) -> (5, -63.3205)
  arc A83 (8, -66.3205) -> (5, -63.3205) centre (5, -66.3205) ccw
  line L106 (-11.6604, -79.514) -> (-17.5653, -85.5935)
  arc A84 (-21, -84.2) -> (-17.5653, -85.5935) centre (-19, -84.2) ccw
  line L107 (-21, -84.2) -> (-21, -78.1205)
  arc A85 (-19, -76.1205) -> (-21, -78.1205) centre (-19, -78.1205) ccw
  line L108 (-19, -76.1205) -> (-13.0951, -76.1205)
  arc A86 (-11.6604, -79.514) -> (-13.0951, -76.1205) centre (-13.0951, -78.1205) ccw
  line L109 (13.0951, -76.1205) -> (19, -76.1205)
  arc A87 (21, -78.1205) -> (19, -76.1205) centre (19, -78.1205) ccw
  line L110 (21, -78.1205) -> (21, -84.2)
  arc A88 (17.5653, -85.5935) -> (21, -84.2) centre (19, -84.2) ccw
  line L111 (17.5653, -85.5935) -> (11.6604, -79.514)
  arc A89 (13.0951, -76.1205) -> (11.6604, -79.514) centre (13.0951, -78.1205) ccw
  line L112 (-13.4347, -89.9523) -> (-1.4347, -77.5976)
  arc A90 (1.4347, -77.5976) -> (-1.4347, -77.5976) centre (0, -78.991) ccw
  line L113 (1.4347, -77.5976) -> (13.4347, -89.9523)
  arc A91 (12, -93.3458) -> (13.4347, -89.9523) centre (12, -91.3458) ccw
  line L114 (12, -93.3458) -> (-12, -93.3458)
  arc A92 (-13.4347, -89.9523) -> (-12, -93.3458) centre (-12, -91.3458) ccw
  line L115 (-23, -57.3205) -> (-23, -5)
  line L116 (-23, -5) -> (23, -5)
  line L117 (23, -5) -> (23, -57.3205)
  line L118 (23, -57.3205) -> (-23, -57.3205)
  line L119 (-70.7899, -5) -> (-47.4446, -5)
  line L120 (-30, -63.3205) -> (-30, -10)
  line L121 (30, -63.3205) -> (30, -28.9838)
  line L122 (42.2983, -5) -> (74.1328, -5)
  dimension "d152" = 7
  dimension "d153" = 7
  dimension "d154" = 6
  dimension "d155" = 13
  constraint perpendicular L115 L116
  constraint horizontal L118
  constraint vertical L117
  constraint horizontal L116
  constraint coincident L57 L119.start
  constraint coincident L94 L119.end
  constraint coincident L59.end L60.start
  constraint coincident L95 L120.end
  constraint coincident L3.end L4.start
  constraint coincident L99 L121.end
  constraint coincident L100 L122.start
  constraint coincident L6 L122.end
  measures "d152" distance of L95 L115
  measures "d153" distance of L99 L117
  measures "d154" distance of L60 L118
  measures "d155" distance of L28 L116
extrude "Extruir7" cut sketch "Boceto8" against normal blind 4.8 contours A0 L5 A1 A75 A77 L101 L121 L122 | A34 L58 A35 L93 A69 A71 L119 L120 | A36 L65 A37 L66 A38 A39 L68 A40 L69 A41 L70 A42 L71 A43 L72 A44 L73 A45 L74 A46 L75 A47 A48 L77 A49 L115 L116 L117 L118